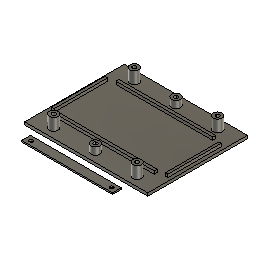
tpl5110-2 v19 (Autodesk Fusion 360 design; units mm, degrees)
Autodesk Fusion 360 part; units mm, degrees
note: some values were not read from the file. Chosen so that the rebuilt part matches the saved one: which bodies a step acts on; which face or edge a step refers to.
box "BoxPrimitive2" add length 48.26 width 95.25 height 2.54 placed x (0, 1, 0) y (-1, 0, 0) z (0, 0, 1) at (95.25, 0, 0) makes body 1
copy_body "CopyPasteBodies1" bodies 1 makes body 2
move_body "Move1" bodies 2 to x (1, 0, 0) y (0, 1, 0) z (0, 0, 1) at (-2.54, -2.54, 0)
move_face "OffsetFaces1" offset 5.08 1 faces at (92.71, 29.6333, 0.8467) on bodies 2
move_face "OffsetFaces2" offset 5.08 1 faces at (64.3467, 45.72, 0.8467) on bodies 2
combine "Combine1" operation cut target body 2 tool bodies 1
scale "Scale1" factors (1.01, 1, 1) about (0, 0, 2.54) bodies 2
box "BoxPrimitive3" add length 86.36 width 106.68 height 12.7 placed x (0, 1, 0) y (-1, 0, 0) z (0, 0, 1) at (102.9392, -8.8534, 2.54) separate body makes body 3
move_body "Move2" bodies 2 to x (1, 0, 0) y (0, 1, 0) z (0, 0, 1) at (0, 0, 25.4)
move_body "Move3" bodies 2 to x (1, 0, 0) y (0, 1, 0) z (0, 0, 1) at (1.778, 11.43, 0)
move_body "Move4" bodies 2 to x (1, 0, 0) y (0, 1, 0) z (0, 0, 1) at (0, -1.016, 0)
copy_body "CopyPasteBodies2" bodies 3 makes body 4
move_body "Move5" bodies 4 to x (1, 0, 0) y (0, 1, 0) z (0, 0, 1) at (2.54, 2.54, 0)
move_body "Move6" bodies 4 to x (1, 0, 0) y (0, 1, 0) z (0, 0, 1) at (0, 0, 2.54)
move_face "OffsetFaces3" offset -5.08 1 faces at (105.4792, 51.2599, 9.3133) on bodies 4
move_face "OffsetFaces4" offset -5.08 1 faces at (32.6659, 80.0466, 9.3133) on bodies 4
combine "Combine2" operation cut target body 3 tool bodies 4
box "BoxPrimitive4" add length 3.81 width 8.89 height 3.81 placed x (0, 1, 0) y (-1, 0, 0) z (0, 0, 1) at (8.89, 0, 0) separate body makes body 5
move_body "Move7" bodies 5 to x (1, 0, 0) y (0, 1, 0) z (0, 0, 1) at (0, 0, 2.54)
move_body "Move8" bodies 5 to x (1, 0, 0) y (0, 1, 0) z (0, 0, 1) at (-0.762, 7.62, 0)
move_body "Move10" bodies 5 to x (1, 0, 0) y (0, 1, 0) z (0, 0, 1) at (0, 0, 2.286)
copy_body "CopyPasteBodies5" bodies 5 makes body 6
move_body "Move11" bodies 6 to x (1, 0, 0) y (0, 1, 0) z (0, 0, 1) at (-0.254, 50.038, 0)
move_body "Move12" bodies 5 to x (1, 0, 0) y (0, 1, 0) z (0, 0, 1) at (-0.254, 0, 0)
copy_body "CopyPasteBodies6" bodies 5 makes body 7
move_body "Move13" bodies 7 to x (1, 0, 0) y (0, 1, 0) z (0, 0, 1) at (92.71, 0, 0)
copy_body "CopyPasteBodies7" bodies 6 makes body 8
move_body "Move14" bodies 8 to x (1, 0, 0) y (0, 1, 0) z (0, 0, 1) at (92.71, 0, 0)
move_body "Move15" bodies 2 to x (1, 0, 0) y (0, 1, 0) z (0, 0, 1) at (0, 0, -22.86)
move_body "Move16" bodies 2 to x (1, 0, 0) y (0, 1, 0) z (0, 0, 1) at (0, 0, 2.54)
combine "Combine3" operation cut target body 2 tool bodies 5 6 7 8 makes body 9 at (98.8356, 26.8393, 5.08) makes body 10 at (63.754, 60.3673, 7.62) makes body 11 at (0.0677, 42.2487, 7.62)
combine "Combine4" operation add target body 3 tool bodies 2 9 10 11
move_body "Move20" bodies 3 to x (1, 0, 0) y (0, 1, 0) z (0, 0, 1) at (0, 0, -2.54)
sketch "Sketch10" plane through (0, 0, 0) normal (0, 0, 1) x (1, 0, 0)
cylinder "CylinderPrimitive5" add diameter 3.2004 height 10.16 placed x (1, 0, 0) y (0, 1, 0) z (0, 0, 1) at (9.4481, -18.7715, 0) separate body makes body 12
cylinder "CylinderPrimitive6" add diameter 7.62 height 11.43 placed x (1, 0, 0) y (0, 1, 0) z (0, 0, 1) at (6.7224, -20.8563, 0) separate body makes body 13
move_body "Move33" bodies 13 to x (1, 0, 0) y (0, 1, 0) z (0, 0, 1) at (2.54, -5.08, 0)
move_face "MoveFace1" by (0, -20.32, 0) 1 faces at (9.4879, -19.3034, 0) on bodies 12
move_body "Move34" bodies 13 to x (1, 0, 0) y (0, 1, 0) z (0, 0, 1) at (0, 7.62, 0)
move_body "Move35" bodies 12 to x (1, 0, 0) y (0, 1, 0) z (0, 0, 1) at (0, 0.762, 0)
move_body "Align1" bodies 13 to x (1, 0, 0) y (0, 1, 0) z (0, 0, 1) at (0.1857, 0.3068, -0.635)
move_body "Move36" bodies 12 to x (1, 0, 0) y (0, 1, 0) z (0, 0, 1) at (0, 0, 5.08)
move_body "Move37" bodies 13 to x (1, 0, 0) y (0, 1, 0) z (0, 0, 1) at (0, 0, -2.032)
move_body "Move38" bodies 13 to x (1, 0, 0) y (0, 1, 0) z (0, 0, 1) at (0, 0, 4.191)
copy_body "CopyPasteBodies18" bodies 12 makes body 14
move_body "Move44" bodies 14 to x (1, 0, 0) y (0, 1, 0) z (0, 0, 1) at (72.39, 0, 0)
copy_body "CopyPasteBodies19" bodies 13 makes body 15
move_body "Move45" bodies 15 to x (1, 0, 0) y (0, 1, 0) z (0, 0, 1) at (72.39, 0, 0)
copy_body "CopyPasteBodies20" bodies 12 makes body 16
move_body "Move46" bodies 16 to x (1, 0, 0) y (0, 1, 0) z (0, 0, 1) at (36.195, 0, 0)
copy_body "CopyPasteBodies21" bodies 13 makes body 17
move_body "Move47" bodies 17 to x (1, 0, 0) y (0, 1, 0) z (0, 0, 1) at (36.195, 0, 0)
move_face "OffsetFaces6" offset -3.81 1 faces at (44.7563, -17.736, 12.954) on bodies 17
move_body "Move48" bodies 12 13 14 15 16 17 to x (1, 0, 0) y (0, 1, 0) z (0, 0, 1) at (3.81, 15.24, 0)
copy_body "CopyPasteBodies22" bodies 15 14 16 17 12 13 makes body 18 makes body 19 makes body 20 makes body 21 makes body 22 makes body 23
move_body "Move49" bodies 18 19 20 21 22 23 to x (1, 0, 0) y (0, 1, 0) z (0, 0, 1) at (0, 69.85, 0)
move_body "Move50" bodies 12 13 14 15 16 17 18 19 20 21 22 23 to x (1, 0, 0) y (0, 1, 0) z (0, 0, 1) at (0, 2.032, 0)
move_body "Move51" bodies 17 to x (1, 0, 0) y (0, 1, 0) z (0, 0, 1) at (0, 0, -1.524)
move_body "Move52" bodies 17 to x (1, 0, 0) y (0, 1, 0) z (0, 0, 1) at (0, 0, 1.27)
move_body "Move53" bodies 21 to x (1, 0, 0) y (0, 1, 0) z (0, 0, 1) at (0, 0, -1.524)
move_body "Move54" bodies 21 to x (1, 0, 0) y (0, 1, 0) z (0, 0, 1) at (0, 0, 1.27)
combine "Combine11" operation cut target body 13 tool bodies 12
combine "Combine12" operation cut target body 15 tool bodies 14
combine "Combine13" operation cut target body 17 tool bodies 16
combine "Combine14" operation cut target body 18 tool bodies 19
combine "Combine15" operation cut target body 21 tool bodies 20
combine "Combine16" operation cut target body 23 tool bodies 22
box "BoxPrimitive6" add length 7.62 width 78.74 height 1.27 placed x (0, 1, 0) y (-1, 0, 0) z (0, 0, 1) at (78.74, -25.4, 0) separate body makes body 24
move_body "Move55" bodies 24 to x (0, 1, 0) y (-1, 0, 0) z (0, 0, 1) at (91.44, -7.62, 0)
move_body "Move56" bodies 24 to x (1, 0, 0) y (0, 1, 0) z (0, 0, 1) at (-2.54, 2.54, 0)
cylinder "CylinderPrimitive7" add diameter 3.2004 height 2.54 placed x (1, 0, 0) y (0, 1, 0) z (0, 0, 1) at (48.26, -22.86, 0) separate body makes body 25
move_body "Move57" bodies 25 to x (1, 0, 0) y (0, 1, 0) z (0, 0, 1) at (62.23, 21.59, 0)
move_body "Move58" bodies 25 to x (1, 0, 0) y (0, 1, 0) z (0, 0, 1) at (0, 0, -0.508)
copy_body "CopyPasteBodies23" bodies 25 makes body 26
move_body "Move59" bodies 26 to x (1, 0, 0) y (0, 1, 0) z (0, 0, 1) at (0, 69.85, 0)
move_body "Move60" bodies 25 26 to x (1, 0, 0) y (0, 1, 0) z (0, 0, 1) at (0, 0.508, 0)
combine "Combine17" operation cut target body 24 tool bodies 25 26
move_body "Move61" bodies 24 to x (0, 1, 0) y (-1, 0, 0) z (0, 0, 1) at (81.28, -139.7, 0)
combine "Combine18" operation add target body 3 tool bodies 13 15 17 18 21 23
box "BoxPrimitive7" add length 4.4264 width 116.84 height 10.16 placed x (0, 1, 0) y (-1, 0, 0) z (0, 0, 1) at (108.4742, -17.78, 0) separate body makes body 27
move_body "Move62" bodies 27 to x (1, 0, 0) y (0, 1, 0) z (0, 0, 1) at (0, 0, 2.54)
move_body "Move63" bodies 27 to x (1, 0, 0) y (0, 1, 0) z (0, 0, 1) at (0, 7.62, 0)
copy_body "CopyPasteBodies24" bodies 27 makes body 28
move_body "Move64" bodies 28 to x (1, 0, 0) y (0, 1, 0) z (0, 0, 1) at (0, 84.582, 0)
copy_body "CopyPasteBodies25" bodies 28 makes body 29
move_body "Move65" bodies 29 to x (0, 1, 0) y (-1, 0, 0) z (0, 0, 1) at (73.2952, -13.7322, 0)
copy_body "CopyPasteBodies26" bodies 29 makes body 30
move_body "Move66" bodies 30 to x (1, 0, 0) y (0, 1, 0) z (0, 0, 1) at (105.918, 0, 0)
move_body "Move67" bodies 29 to x (1, 0, 0) y (0, 1, 0) z (0, 0, 1) at (0.508, 0, 0)
move_body "Move68" bodies 30 to x (1, 0, 0) y (0, 1, 0) z (0, 0, 1) at (-0.254, 0, 0)
combine "Combine19" operation cut target body 3 tool bodies 27 28 29 30
move_body "Move69" bodies 24 to x (1, 0, 0) y (0, 1, 0) z (0, 0, 1) at (0, 10.16, 0)
cylinder "CylinderPrimitive8" add diameter 3.302 height 7.62 placed x (1, 0, 0) y (0, 1, 0) z (0, 0, 1) at (22.5704, -34.514, 0) separate body makes body 31
move_body "Move71" bodies 31 to x (1, 0, 0) y (0, 1, 0) z (0, 0, 1) at (-10.16, 33.02, 0)
move_body "Move72" bodies 31 to x (1, 0, 0) y (0, 1, 0) z (0, 0, 1) at (0.889, 0.635, 6.35)
copy_body "CopyPasteBodies28" bodies 31 makes body 32
move_body "Move73" bodies 32 to x (1, 0, 0) y (0, 1, 0) z (0, 0, 1) at (72.39, 0, 0)
copy_body "CopyPasteBodies29" bodies 31 makes body 33
move_body "Move74" bodies 33 to x (1, 0, 0) y (0, 1, 0) z (0, 0, 1) at (0, 69.85, 0)
copy_body "CopyPasteBodies30" bodies 33 makes body 34
move_body "Move75" bodies 34 to x (1, 0, 0) y (0, 1, 0) z (0, 0, 1) at (72.39, 0, 0)
copy_body "CopyPasteBodies31" bodies 31 makes body 35
move_body "Move76" bodies 35 to x (1, 0, 0) y (0, 1, 0) z (0, 0, 1) at (36.068, 0, -5.08)
copy_body "CopyPasteBodies32" bodies 35 makes body 36
move_body "Move77" bodies 36 to x (1, 0, 0) y (0, 1, 0) z (0, 0, 1) at (0, 69.85, 0)
combine "Combine20" operation cut target body 3 tool bodies 31 32 33 34 35 36
named bodies: "battery_barrier1", "base", "basecutout", "barriercut1", "barriercut2", "barriercut1 (1)", "barriercut3", "barriercut2 (1)", "battery_barrier2", "battery_barrier3", "battery_barrier4", "strap"
